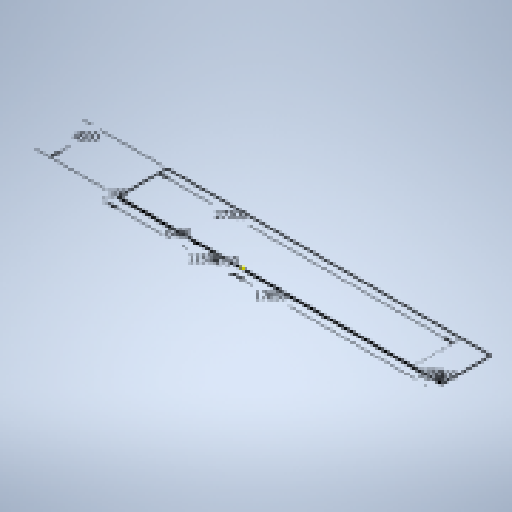
# Autodesk Inventor part: NDM-VOS dummy FLOOR
Saved by Autodesk Inventor 2025 (Build 290162010, 162A)
## iProperties
Created: 2024-10-13
Part Number: NDM-VOS dummy FLOOR
Material: Generic
Document SubType Name: Modeling
Designer: admin
Density: 1 g/cm^3
Appearance: Default
Author: admin
Autodesk Inventor part; units mm, degrees
ref_plane "YZ Plane" through (0, 0, 0) normal (1, 0, 0) x (0, 1, 0)
ref_plane "XZ Plane" through (0, 0, 0) normal (0, 1, 0) x (-1, 0, 0)
ref_plane "XY Plane" through (0, 0, 0) normal (0, 0, 1) x (1, 0, 0)
sketch "Sketch1" plane through (0, 0, 0) normal (0, 0, 1) x (1, 0, 0)
  line L0 (-11500, 4500) -> (15700, 4500)
  line L1 (15700, 4500) -> (15700, 0) construction
  line L2 (15700, 0) -> (-11500, 0)
  line L3 (-11500, 0) -> (-11500, 4500)
  line L4 (18150, 0) -> (17850, 0)
  line L5 (17850, 0) -> (17850, 500)
  line L6 (17850, 500) -> (18150, 500)
  line L7 (18150, 500) -> (18150, 0)
  line L8 (15700, 0) -> (18470, 0)
  line L9 (18470, 0) -> (18470, 4500)
  line L10 (18470, 4500) -> (15700, 4500)
  line L11 (-11500, 0) -> (-11500, -100)
  line L12 (-11500, -100) -> (18470, -100)
  line L13 (18470, -100) -> (18470, 0)
  line L14 (-5100, 0) -> (-5100, -100)
  line L15 (-350, 0) -> (-350, -100)
  line L16 (11850, 0) -> (11850, 500)
  line L17 (12150, 0) -> (11850, 0)
  line L18 (11850, 500) -> (12150, 500)
  line L19 (12150, 500) -> (12150, 0)
  line L20 (5850, 0) -> (5850, 500)
  line L21 (6150, 0) -> (5850, 0)
  line L22 (5850, 500) -> (6150, 500)
  line L23 (6150, 500) -> (6150, 0)
  line L24 (-150, 0) -> (-150, 500)
  line L25 (150, 0) -> (-150, 0)
  line L26 (-150, 500) -> (150, 500)
  line L27 (150, 500) -> (150, 0)
  line L28 (-6150, 0) -> (-6150, 500)
  line L29 (-5850, 0) -> (-6150, 0)
  line L30 (-6150, 500) -> (-5850, 500)
  line L31 (-5850, 500) -> (-5850, 0)
  line L32 (-11500, 0) -> (-11200, 0)
  line L33 (-11200, 0) -> (-11200, 500)
  line L34 (-11200, 500) -> (-11500, 500)
  line L35 (-11500, 500) -> (-11500, 0)
  point P0 (0, 0)
  dimension "d0" = 4500
  dimension "d1" = 27200
  dimension "d2" = 300
  dimension "d3" = 500
  dimension "d4" = 11500
  dimension "d5" = 17850
  dimension "d6" = 2770
  dimension "d7" = 100
  dimension "d8" = 4750
  dimension "d9" = 6400
  dimension "d16" = 6000
  dimension "d21" = 5350
  constraints: 72 end point, 9 perpendicular, 7 point on line, 6 parallel, 5 horizontal, 2 equal length, 1 vertical, 32 other
  measures "d0" distance of L2.end L0.start
  measures "d1" distance of L0.start L0.end
  measures "d2" distance of L5.end L6.end
  measures "d3" distance of L4.end L5.end
  measures "d4" distance from line of point (0, 0) L3
  measures "d5" distance of point (0, 0) L4.end
  measures "d6" distance of L1.end L8.end
  measures "d7" distance between parallel lines of L2 L12
  measures "d8" distance between parallel lines of L15 L14
  measures "d9" distance between parallel lines of L14 L11
  measures "d16" distance of L5.end L16.end
  measures "d21" distance between parallel lines of L28 L35
extrude "Extrusion1" add sketch "Sketch1" against normal blind 10 contours L0 L10 L9 L8 L7 L6 L5 L2 L19 L18 L16 L23 L22 L20 L27 L26 L24 L31 L30 L28 L33 L34 L3 | L34 L33 L2 L3 | L13 L12 L15 L2 L8 L4 | L4 L5 L6 L7 | L28 L30 L31 L2 | L2 L16 L18 L19 | L24 L26 L27 L2 | L2 L20 L22 L23
extrude "Extrusion2" add sketch "Sketch1" along normal blind 4000 separate body contours L34 L33 L2 L3 | L4 L5 L6 L7 | L28 L30 L31 L2 | L2 L16 L18 L19 | L24 L26 L27 L2 | L2 L20 L22 L23
extrude "Extrusion3" add sketch "Sketch1" along normal blind 300 separate body contours L2 L14 L12 L11 | L13 L12 L15 L2 L8 L4
body "Solid1"
